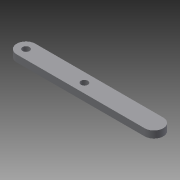
# Autodesk Inventor part: leg
Saved by Autodesk Inventor 2014 (Build 180170000, 170)
## iProperties
Created: 2015-03-09
Part Number: leg
Material: 一般
Document SubType Name: Modeling
Designer: Hideyuki Takei
Density: 1 g/cm^3
Appearance: 既定
Author: Hideyuki Takei
Autodesk Inventor part; units mm, degrees
ref_plane "YZ Plane" through (0, 0, 0) normal (1, 0, 0) x (0, 1, 0)
ref_plane "XZ Plane" through (0, 0, 0) normal (0, 1, 0) x (-1, 0, 0)
ref_plane "XY Plane" through (0, 0, 0) normal (0, 0, 1) x (1, 0, 0)
sketch "スケッチ1" plane through (0, 0, 0) normal (0, 0, 1) x (1, 0, 0)
  line L0 (0, 0) -> (55, 0) construction
  line L1 (0, -4) -> (55, -4)
  line L2 (55, 4) -> (0, 4)
  arc A0 (0, 4) -> (0, -4) centre (0, 0) ccw
  arc A1 (55, -4) -> (55, 4) centre (55, 0) ccw
  circle A2 centre (0, 0) radius 1.5
  circle A3 centre (25.1, 0) radius 1.5
  point P0 (27.5, 0)
  dimension "d0" = 4
  dimension "d1" = 55
  dimension "d2" = 3
  dimension "d3" = 3
  dimension "d4" = 25.1
  constraints: 8 end point, 4 centre point, 4 point on circle, 4 tangent, 1 coincident, 1 horizontal, 1 midpoint, 1 parallel, 1 point on line
  measures "d0" radius of A0
  measures "d1" distance of L0.start L0.end
  measures "d2" diameter of A2
  measures "d3" diameter of A3
  measures "d4" distance of L0.start A3.centre
extrude "押し出し1" add sketch "スケッチ1" along normal blind 3
